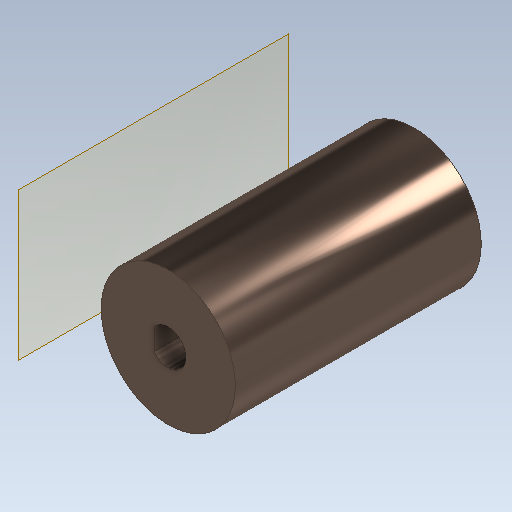
# Autodesk Inventor part: ballscrew coupler
Saved by Autodesk Inventor 2020 (Build 240168000, 168)
## iProperties
Created: 2020-07-30
Part Number: ballscrew coupler
Material: Steel, Mild
Document SubType Name: Modeling
Designer: Vikki
Mass: 266.884 g
Surface Area: 83.1233 cm^2
Volume: 33.9979 cm^3
Density: 7.85 g/cm^3
Appearance: Gunmetal - Antique Polished
Author: Vikki
Autodesk Inventor part; units mm, degrees
ref_plane "XZ Plane" through (0, 0, 0) normal (0, 1, 0) x (-1, 0, 0)
ref_plane "XY Plane" through (0, 0, 0) normal (0, 0, 1) x (1, 0, 0)
sketch "Sketch1" plane through (0, 0, 0) normal (0, 0, 1) x (1, 0, 0)
  line L0 (-5, 6.245) -> (-5, -6.245) projected
  arc A0 (-5, -6.245) -> (-5, 6.245) centre (0, 0) ccw projected
  circle A1 centre (0, 0) radius 15
  dimension "d0" = 30
  constraints: 1 centre point, 1 coincident
  measures "d0" diameter of A1
extrude "Extrusion1" add sketch "Sketch1" against normal blind 20
sketch "Sketch2" plane through (0, 0, 0) normal (0, 0, 1) x (1, 0, 0)
  circle A0 centre (0, 0) radius 15 projected
extrude "Extrusion2" add sketch "Sketch2" along normal blind 15
sketch "Sketch3" plane through (0, 0, 15) normal (0, 0, 1) x (1, 0, 0)
  line L0 (-3.175, -2.433) -> (-3.175, 2.433) projected
  arc A0 (-3.175, -2.433) -> (-3.175, 2.433) centre (0, 0) ccw projected
  circle A1 centre (0, 0) radius 15 projected
extrude "Extrusion3" add sketch "Sketch3" along normal blind 20
ref_plane "Work Plane1" through (-30.75, 0, 0) normal (1, 0, 0) x (0, 1, 0)
sketch "Sketch4" plane through (-30.75, 0, 0) normal (1, 0, 0) x (0, 1, 0)
  line L0 (15, 35) -> (-15, 35) projected
  line L1 (-15, -20) -> (15, -20) projected
  line L2 (-15, 35) -> (-15, -20) projected
  line L3 (15, 35) -> (15, -20) projected
  circle A0 centre (0, -10) radius 3
  circle A1 centre (0, 20) radius 2
  point P0 (0, 0)
  dimension "d8" = 4
  dimension "d9" = 6
  dimension "d10" = 10
  dimension "d11" = 15
  constraints: 2 centre point, 2 vertical alignment
  measures "d8" diameter of A1
  measures "d9" diameter of A0
  measures "d10" distance from line of L1 A0.centre
  measures "d11" distance from line of L0 A1.centre
extrude "Extrusion4" cut sketch "Sketch4" along normal up to surface (30.75 mm away) contours A0 | A1
thread "Thread1" size "M6x1" class "6H" standard "ANSI Metric M Profile" length 60
thread "Thread2" size "M4x0.7" class "6H" standard "ANSI Metric M Profile" length 60
body "Solid1"
